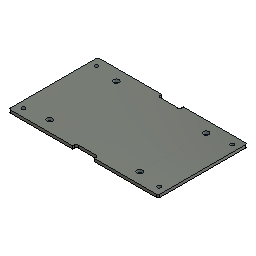
Three Chanel Board v4 (Autodesk Fusion 360 design; units mm, degrees)
Autodesk Fusion 360 part; units mm, degrees
sketch "Sketch1" plane through (0, 0, 0) normal (0, 1, 0) x (1, 0, 0)
  line L0 (41.5, 24.75) -> (-41.5, 24.75)
  line L1 (-41.5, 24.75) -> (-41.5, -24.75)
  line L2 (-41.5, -24.75) -> (41.5, -24.75)
  line L3 (41.5, -24.75) -> (41.5, 24.75)
  line L4 (41.5, 24.75) -> (-41.5, -24.75) construction
  line L5 (-41.5, 24.75) -> (41.5, -24.75) construction
  line L6 (6, 26.75) -> (-6, 26.75)
  line L7 (-6, 26.75) -> (-6, 22.75)
  line L8 (-6, 22.75) -> (6, 22.75)
  line L9 (6, 22.75) -> (6, 26.75)
  line L10 (6, 26.75) -> (-6, 22.75) construction
  line L11 (-6, 26.75) -> (6, 22.75) construction
  line L12 (6, -26.75) -> (-6, -26.75)
  line L13 (-6, -26.75) -> (-6, -22.75)
  line L14 (-6, -22.75) -> (6, -22.75)
  line L15 (6, -22.75) -> (6, -26.75)
  point P0 (0, 24.75)
  dimension "d1" = 83
  dimension "d2" = 49.5
  dimension "d3" = 12
  dimension "d4" = 4
  constraint horizontal L0
  constraint perpendicular L0 L1
  constraint parallel L0 L2
  constraint parallel L1 L3
  constraint coincident L4 origin
  constraint coincident L5 origin
  constraint horizontal L6
  constraint perpendicular L6 L7
  constraint parallel L6 L8
  constraint parallel L7 L9
  constraint coincident L10 P0
  constraint coincident L11 P0
  constraint midpoint L0 P0
  measures "d1" distance of L1.end L2.end
  measures "d2" distance of L0.end L1.end
  measures "d3" distance of L7.end L8.end
  measures "d4" distance of L6.end L7.end
extrude "Extrude1" add sketch "Sketch1" along normal blind 1.6 contours L0 L1 L2 L3 L7 L8 L9 L13 L14 L15
fillet "Fillet1" radius 1 4 edges at (6, 0.8, 22.75) (-6, 0.8, 22.75) (6, 0.8, -22.75) (-6, 0.8, -22.75)
fillet "Fillet2" radius 1 4 edges at (-41.5, 0.8, -24.75) (-41.5, 0.8, 24.75) (41.5, 0.8, 24.75) (41.5, 0.8, -24.75)
sketch "Sketch2" plane through (0, 1.6, 0) normal (0, 1, 0) x (-1, 0, 0)
  arc A0 (-41.5, -23.75) -> (-40.5, -24.75) centre (-40.5, -23.75) ccw
  line L0 (-40.5, -24.75) -> (-6, -24.75)
  line L1 (-6, -24.75) -> (-6, -23.75)
  arc A1 (-5, -22.75) -> (-6, -23.75) centre (-5, -23.75) ccw
  line L2 (-5, -22.75) -> (5, -22.75)
  arc A2 (6, -23.75) -> (5, -22.75) centre (5, -23.75) ccw
  line L3 (6, -23.75) -> (6, -24.75)
  line L4 (6, -24.75) -> (40.5, -24.75)
  arc A3 (40.5, -24.75) -> (41.5, -23.75) centre (40.5, -23.75) ccw
  line L5 (41.5, -23.75) -> (41.5, 23.75)
  arc A4 (41.5, 23.75) -> (40.5, 24.75) centre (40.5, 23.75) ccw
  line L6 (40.5, 24.75) -> (6, 24.75)
  line L7 (6, 24.75) -> (6, 23.75)
  arc A5 (5, 22.75) -> (6, 23.75) centre (5, 23.75) ccw
  line L8 (5, 22.75) -> (-5, 22.75)
  arc A6 (-6, 23.75) -> (-5, 22.75) centre (-5, 23.75) ccw
  line L9 (-6, 23.75) -> (-6, 24.75)
  line L10 (-6, 24.75) -> (-40.5, 24.75)
  arc A7 (-40.5, 24.75) -> (-41.5, 23.75) centre (-40.5, 23.75) ccw
  line L11 (-41.5, 23.75) -> (-41.5, -23.75)
  circle A8 centre (25, 18.5) radius 1.5
  circle A9 centre (25, -18.5) radius 1.5
  circle A10 centre (-25, -18.5) radius 1.5
  circle A11 centre (-25, 18.5) radius 1.5
  dimension "d11" = 50
  dimension "d12" = 37
  dimension "d13" = 3
  dimension "d14" = 3
  dimension "d15" = 3
  dimension "d16" = 3
  measures "d11" distance of A9.centre A10.centre
  measures "d12" distance of A10.centre A11.centre
  measures "d13" diameter of A8
  measures "d14" diameter of A9
  measures "d15" diameter of A10
  measures "d16" diameter of A11
extrude "Extrude2" cut sketch "Sketch2" against normal blind 6 contours A8 | A9 | A10 | A11
sketch "Sketch3" plane through (0, 1.6, 0) normal (0, 1, 0) x (-1, 0, 0)
  circle A0 centre (25, 18.5) radius 1.5
  circle A1 centre (-25, 18.5) radius 1.5
  circle A2 centre (25, -18.5) radius 1.5
  circle A3 centre (-25, -18.5) radius 1.5
  arc A4 (-41.5, -23.75) -> (-40.5, -24.75) centre (-40.5, -23.75) ccw
  line L0 (-40.5, -24.75) -> (-6, -24.75)
  line L1 (-6, -24.75) -> (-6, -23.75)
  arc A5 (-5, -22.75) -> (-6, -23.75) centre (-5, -23.75) ccw
  line L2 (-5, -22.75) -> (5, -22.75)
  arc A6 (6, -23.75) -> (5, -22.75) centre (5, -23.75) ccw
  line L3 (6, -23.75) -> (6, -24.75)
  line L4 (6, -24.75) -> (40.5, -24.75)
  arc A7 (40.5, -24.75) -> (41.5, -23.75) centre (40.5, -23.75) ccw
  line L5 (41.5, -23.75) -> (41.5, 23.75)
  arc A8 (41.5, 23.75) -> (40.5, 24.75) centre (40.5, 23.75) ccw
  line L6 (40.5, 24.75) -> (6, 24.75)
  line L7 (6, 24.75) -> (6, 23.75)
  arc A9 (5, 22.75) -> (6, 23.75) centre (5, 23.75) ccw
  line L8 (5, 22.75) -> (-5, 22.75)
  arc A10 (-6, 23.75) -> (-5, 22.75) centre (-5, 23.75) ccw
  line L9 (-6, 23.75) -> (-6, 24.75)
  line L10 (-6, 24.75) -> (-40.5, 24.75)
  arc A11 (-40.5, 24.75) -> (-41.5, 23.75) centre (-40.5, 23.75) ccw
  line L11 (-41.5, 23.75) -> (-41.5, -23.75)
  circle A12 centre (37.75, 20.3) radius 1
  circle A13 centre (37.75, -20.3) radius 1
  circle A14 centre (-37.75, 20.3) radius 1
  circle A15 centre (-37.75, -20.3) radius 1
  dimension "d19" = 75.5
  dimension "d20" = 40.6
  dimension "d21" = 2
  dimension "d22" = 2
  dimension "d23" = 2
  dimension "d24" = 2
  measures "d19" distance of A13.centre A15.centre
  measures "d20" distance of A14.centre A15.centre
  measures "d21" diameter of A12
  measures "d22" diameter of A13
  measures "d23" diameter of A14
  measures "d24" diameter of A15
extrude "Extrude3" cut sketch "Sketch3" against normal blind 2 contours A12 | A13 | A14 | A15
sketch "Sketch4" plane through (0, 1.6, 0) normal (0, 1, 0) x (-1, 0, 0)
  circle A0 centre (37.75, 20.3) radius 1
  circle A1 centre (37.75, -20.3) radius 1
  circle A2 centre (-37.75, 20.3) radius 1
  circle A3 centre (-37.75, -20.3) radius 1
  circle A4 centre (25, 18.5) radius 1.5
  circle A5 centre (-25, 18.5) radius 1.5
  circle A6 centre (25, -18.5) radius 1.5
  circle A7 centre (-25, -18.5) radius 1.5
  arc A8 (-41.5, -23.75) -> (-40.5, -24.75) centre (-40.5, -23.75) ccw
  line L0 (-40.5, -24.75) -> (-6, -24.75)
  line L1 (-6, -24.75) -> (-6, -23.75)
  arc A9 (-5, -22.75) -> (-6, -23.75) centre (-5, -23.75) ccw
  line L2 (-5, -22.75) -> (5, -22.75)
  arc A10 (6, -23.75) -> (5, -22.75) centre (5, -23.75) ccw
  line L3 (6, -23.75) -> (6, -24.75)
  line L4 (6, -24.75) -> (40.5, -24.75)
  arc A11 (40.5, -24.75) -> (41.5, -23.75) centre (40.5, -23.75) ccw
  line L5 (41.5, -23.75) -> (41.5, 23.75)
  arc A12 (41.5, 23.75) -> (40.5, 24.75) centre (40.5, 23.75) ccw
  line L6 (40.5, 24.75) -> (6, 24.75)
  line L7 (6, 24.75) -> (6, 23.75)
  arc A13 (5, 22.75) -> (6, 23.75) centre (5, 23.75) ccw
  line L8 (5, 22.75) -> (-5, 22.75)
  arc A14 (-6, 23.75) -> (-5, 22.75) centre (-5, 23.75) ccw
  line L9 (-6, 23.75) -> (-6, 24.75)
  line L10 (-6, 24.75) -> (-40.5, 24.75)
  arc A15 (-40.5, 24.75) -> (-41.5, 23.75) centre (-40.5, 23.75) ccw
  line L11 (-41.5, 23.75) -> (-41.5, -23.75)
